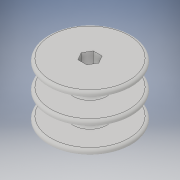
# Autodesk Inventor part: spool
Saved by Autodesk Inventor 2019.3 (Build 233278000, 278)
## iProperties
Created: 2019-02-25
Part Number: spool
Material: Generic
Document SubType Name: Modeling
Designer: steele
Density: 1 g/cm^3
Appearance: Default
Author: steele
Autodesk Inventor part; units mm, degrees
ref_plane "YZ Plane" through (0, 0, 0) normal (1, 0, 0) x (0, 1, 0)
ref_plane "XZ Plane" through (0, 0, 0) normal (0, 1, 0) x (-1, 0, 0)
ref_plane "XY Plane" through (0, 0, 0) normal (0, 0, 1) x (1, 0, 0)
sketch "Sketch1" plane through (0, 0, 0) normal (1, 0, 0) x (0, 1, 0)
  line L0 (0, 0) -> (0, -35.56)
  line L1 (2.54, -38.1) -> (2.54, -38.1)
  line L2 (5.08, -35.56) -> (5.08, -15.24)
  line L3 (7.62, -12.7) -> (20.32, -12.7)
  line L4 (22.86, -15.24) -> (22.86, -35.56)
  line L5 (25.4, -38.1) -> (25.4, -38.1)
  line L6 (27.94, -35.56) -> (27.94, -15.24)
  line L7 (30.48, -12.7) -> (43.18, -12.7)
  line L8 (45.72, -15.24) -> (45.72, -35.56)
  line L9 (48.26, -38.1) -> (48.26, -38.1)
  line L10 (50.8, -35.56) -> (50.8, 0)
  line L11 (0, 0) -> (50.8, 0)
  arc A0 (48.26, -38.1) -> (50.8, -35.56) centre (48.26, -35.56) ccw
  arc A1 (45.72, -35.56) -> (48.26, -38.1) centre (48.26, -35.56) ccw
  arc A2 (25.4, -38.1) -> (27.94, -35.56) centre (25.4, -35.56) ccw
  arc A3 (22.86, -35.56) -> (25.4, -38.1) centre (25.4, -35.56) ccw
  arc A4 (2.54, -38.1) -> (5.08, -35.56) centre (2.54, -35.56) ccw
  arc A5 (0, -35.56) -> (2.54, -38.1) centre (2.54, -35.56) ccw
  arc A6 (45.72, -15.24) -> (43.18, -12.7) centre (43.18, -15.24) ccw
  arc A7 (30.48, -12.7) -> (27.94, -15.24) centre (30.48, -15.24) ccw
  arc A8 (22.86, -15.24) -> (20.32, -12.7) centre (20.32, -15.24) ccw
  arc A9 (7.62, -12.7) -> (5.08, -15.24) centre (7.62, -15.24) ccw
  point P0 (45.72, -38.1)
  point P1 (50.8, -38.1)
  dimension "d0" = 50.8
  dimension "d1" = 5.08
  dimension "d2" = 12.7
  dimension "d3" = 38.1
  dimension "d4" = 2.54
  dimension "d5" = 2.54
  constraints: 24 end point, 20 point on circle, 20 tangent, 10 centre point, 8 equal radius, 6 perpendicular, 6 point on line, 5 collinear, 1 horizontal, 1 parallel, 1 vertical
  measures "d0" distance between parallel lines of L10 L0
  measures "d1" distance of point (45.72, -38.1) point (50.8, -38.1)
  measures "d2" distance between parallel lines of L3 L11
  measures "d3" distance between parallel lines of L1 L11
  measures "d4" radius of A0
  measures "d5" radius of A6
revolve "Revolution1" add sketch "Sketch1" angle 360 about axis through (0, 0, 0) along (0, 1, 0)
sketch "Sketch2" plane through (0, 50.8, 0) normal (0, 1, 0) x (1, 0, 0)
  line L0 (8.0656, 0) -> (4.0328, -6.985)
  line L1 (4.0328, -6.985) -> (-4.0328, -6.985)
  line L2 (-4.0328, -6.985) -> (-8.0656, 0)
  line L3 (-8.0656, 0) -> (-4.0328, 6.985)
  line L4 (-4.0328, 6.985) -> (4.0328, 6.985)
  line L5 (4.0328, 6.985) -> (8.0656, 0)
  point P0 (0, 0)
  point P1 (0, 0)
  dimension "d8" = 13.97
  constraints: 12 end point, 1 coincident, 1 horizontal, 13 other
  measures "d8" distance between parallel lines of L1 L4
extrude "Extrusion1" cut sketch "Sketch2" against normal through all
sketch "Sketch4" plane through (0, 0, 0) normal (1, 0, 0) x (0, 1, 0)
  circle A0 centre (36.83, 8.89) radius 1.75
  circle A1 centre (13.97, 8.89) radius 1.75
  line L0 (5.08, 35.56) -> (5.08, -35.56) projected
  line L1 (45.72, 35.56) -> (45.72, -35.56) projected
  line L2 (50.8, 0) -> (0, 0) projected
  dimension "d17" = 8.89
  dimension "d18" = 8.89
  dimension "d19" = 3.5
  dimension "d20" = 8.89
  dimension "d21" = 8.89
  constraints: 2 centre point, 1 equal radius
  measures "d17" distance from line of A1.centre L0
  measures "d18" distance from line of A0.centre L1
  measures "d19" diameter of A0
  measures "d20" distance from line of A1.centre L2
  measures "d21" distance from line of A0.centre L2
extrude "Extrusion3" cut sketch "Sketch4" along normal through all both and the other way through all
equation "\"d0\" = spoolHeight"
equation "\"d1\" = supportChannels"
equation "\"d2\" = spoolInteriroRadius"
equation "\"d3\" = spoolExteriorRadius"
equation "\"d4\" = spoolFiletRadius"
equation "\"d5\" = spoolFiletRadius"
equation "\"d8\" = hexDiameter"
equation "\"d19\" = holeForString"
equation "\"holeForString\" = stringDiameter + clearanceForString"
equation "\"stringDiameter\" = 3"
equation "\"clearanceForString\" = 0.5"
equation "\"spoolHeight\" = 50.8"
equation "\"hexShaftDiameter\" = 12.7"
equation "\"clearanceForHexShaft\" = 1.27"
equation "\"hexDiameter\" = hexShaftDiameter + clearanceForHexShaft"
equation "\"supportChannels\" = 5.08"
equation "\"spoolInteriorDiameter\" = 25.4"
equation "\"spoolInteriroRadius\" = 0.5 * spoolInteriorDiameter"
equation "\"spoolExteriorDiameter\" = 76.2"
equation "\"spoolExteriorRadius\" = 0.5 * spoolExteriorDiameter"
equation "\"spoolFiletRadius\" = 0.5 * supportChannels"
equation "\"holeCenter\" = 25.4"
body "Solid1"
